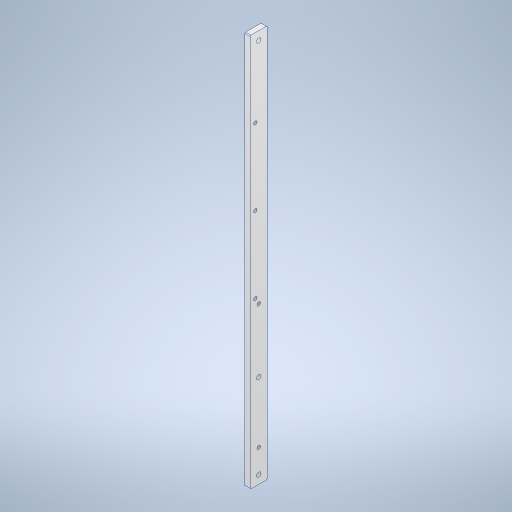
# Autodesk Inventor part: Door Aluminum Bars
Saved by Autodesk Inventor 2024 (Build 280153000, 153)
## iProperties
Created: 2024-08-28
Part Number: Door Aluminum Bars
Material: Aluminum 6061
Document SubType Name: Modeling
Designer: Ishaan
Density: 2.7 g/cm^3
Appearance: Aluminum - Flat
Mass: 157.839 g
Surface Area: 250.43 cm^2
Volume: 58.4588 cm^3
Author: Ishaan
Autodesk Inventor part; units mm, degrees
ref_plane "YZ Plane" through (0, 0, 0) normal (1, 0, 0) x (0, 1, 0)
ref_plane "XZ Plane" through (0, 0, 0) normal (0, 1, 0) x (-1, 0, 0)
ref_plane "XY Plane" through (0, 0, 0) normal (0, 0, 1) x (1, 0, 0)
sketch "Sketch1" plane through (0, 0, 0) normal (1, 0, 0) x (0, 1, 0)
  line L0 (-232.5, -10) -> (232.5, -10)
  line L1 (232.5, -10) -> (232.5, 10)
  line L2 (232.5, 10) -> (-232.5, 10)
  line L3 (-232.5, 10) -> (-232.5, -10)
  line L4 (-232.5, -10) -> (232.5, 10) construction
  line L5 (232.5, -10) -> (-232.5, 10) construction
  point P0 (0, 0)
  dimension "d0" = 465
  dimension "d1" = 20
  constraints: 12 end point, 2 midpoint, 2 parallel, 1 horizontal, 1 perpendicular
  measures "d0" distance of L2.end L1.end
  measures "d1" distance of L1.end L0.end
extrude "Extrusion1" add sketch "Sketch1" along normal blind 6.35
sketch "Sketch2" plane through (6.35, 0, 0) normal (1, 0, 0) x (0, 0, -1)
  line L0 (10, 232.5) -> (-10, 232.5) projected
  line L1 (-10, 232.5) -> (-10, -232.5) projected
  line L2 (-10, -232.5) -> (10, -232.5) projected
  line L3 (10, -232.5) -> (10, 232.5) projected
  point P0 (0, 0)
  point P1 (0, 222.5)
  point P2 (0, 232.5)
  point P3 (0, -222.5)
  point P4 (0, -122.5)
  dimension "d4" = 10
  dimension "d5" = 10
  dimension "d6" = 100
  constraints: 3 vertical alignment, 1 midpoint
  measures "d4" distance from line of point (0, 222.5) L0
  measures "d5" distance from line of L2 point (0, -222.5)
  measures "d6" distance of point (0, -222.5) point (0, -122.5)
hole "Hole1" at (6.35, 222.5, 0) at (6.35, -222.5, 0) at (6.35, -122.5, 0) direction (-1, 0, 0) diameter 5.3 end through all
sketch "Sketch3" plane through (6.35, 0, 0) normal (1, 0, 0) x (0, 0, -1)
  circle A0 centre (0, -122.5) radius 2.65 projected
  circle A1 centre (0, -222.5) radius 2.65 projected
  circle A2 centre (0, 222.5) radius 2.65 projected
  line L0 (10, 232.5) -> (-10, 232.5) projected
  line L1 (-10, 232.5) -> (-10, -232.5) projected
  line L2 (-10, -232.5) -> (10, -232.5) projected
  line L3 (10, -232.5) -> (10, 232.5) projected
  point P0 (0, 0)
  point P1 (0, -194.5)
  point P2 (0, -47.5)
  dimension "d14" = 72
  dimension "d22" = 147
  constraints: 2 vertical alignment
  measures "d14" distance of point (0, -194.5) A0.centre
  measures "d22" distance of point (0, -194.5) point (0, -47.5)
hole "Hole2" at (6.35, -194.5, 0) at (6.35, -47.5, 0) direction (-1, 0, 0) diameter 4.134 end through all thread size "M5x0.8" class "6H" standard "ANSI Metric M Profile"
fillet "Fillet1" radius 1 4 edges at (3.175, -232.5, 10) (3.175, -232.5, -10) (3.175, 232.5, 10) (3.175, 232.5, -10)
sketch "Sketch4" plane through (6.35, 0, 0) normal (1, 0, 0) x (0, 0, -1)
  circle A0 centre (0, 222.5) radius 2.65 projected
  line L0 (-4, 140) -> (-4, -40) construction
  line L1 (-10, 231.5) -> (-10, -231.5) projected
  line L2 (0, 222.5) -> (0, -122.5) construction
  circle A1 centre (0, -122.5) radius 2.65 projected
  point P0 (0, 0)
  point P1 (-4, 50)
  point P2 (0, 50)
  point P3 (-4, 50)
  dimension "d24" = 180
  dimension "d25" = 6
  constraints: 4 coincident, 4 end point, 2 midpoint, 2 vertical, 1 horizontal alignment
  measures "d24" distance of L0.start L0.end
  measures "d25" distance between parallel lines of L0 L1
hole "Hole3" at (6.35, 140, 4) at (6.35, 50, 4) at (6.35, -40, 4) direction (-1, 0, 0) diameter 4.134 end through all thread size "M5x0.8" class "6H" standard "ANSI Metric M Profile"
body "Solid1"
